# Autodesk Inventor part: SN74LV244A
Saved by Autodesk Inventor 2015 SP1 (Build 190203100, 203)
## iProperties
Created: 2015-06-25
Part Number: SN74LV244A
Material: Generic
Document SubType Name: Modeling
Designer: Patrick
Density: 1 g/cm^3
Appearance: TSSOP20, SN74LV244A
Author: Patrick
Autodesk Inventor part; units mm, degrees
ref_plane "YZ Plane" through (0, 0, 0) normal (1, 0, 0) x (0, 1, 0)
ref_plane "XZ Plane" through (0, 0, 0) normal (0, 1, 0) x (-1, 0, 0)
ref_plane "XY Plane" through (0, 0, 0) normal (0, 0, 1) x (1, 0, 0)
sketch "TSSOP20, SN74LV244A_143" plane through (0, 0, 0) normal (0, 0, 1) x (1, 0, 0)
  line L0 (-3.886, -3.35) -> (-3.886, 3.756)
  line L1 (-3.886, 3.756) -> (3.7, 3.756)
  line L2 (3.7, 3.756) -> (3.7, -3.35)
  line L3 (3.7, -3.35) -> (-3.886, -3.35)
  constraints: 8 end point
extrude "Extrusion1" add sketch "TSSOP20, SN74LV244A_143" along normal blind 1
body "Solid1"
